Autodesk Fusion 360 part; units mm, degrees
(part 7 of 9)
  spline S37 degree 5 poles (66.3384, -8.5688) (66.3471, -8.5734) (66.3642, -8.5827) (66.3895, -8.5974) (66.4225, -8.6182) (66.4628, -8.6459) (66.5024, -8.6748) (66.5415, -8.7044) (66.5803, -8.7345) (66.6191, -8.7648) (66.6576, -8.7955) (66.6959, -8.8265) (66.7339, -8.858) (66.7716, -8.8901) (66.8088, -8.9228) (66.8458, -8.956) (66.8824, -8.9896) (66.9188, -9.0237) (66.955, -9.0581) (66.9909, -9.0927) (67.0267, -9.1277) (67.0622, -9.1631) (67.0975, -9.1987) (67.1325, -9.2348) (67.1673, -9.2712) (67.2019, -9.3079) (67.2362, -9.3449) (67.2704, -9.3822) (67.3043, -9.4198) (67.338, -9.4577) (67.3716, -9.4959) (67.4049, -9.5344) (67.438, -9.5731) (67.4709, -9.6121) (67.5036, -9.6514) (67.5361, -9.6909) (67.5684, -9.7307) (67.6005, -9.7708) (67.6324, -9.8111) (67.6641, -9.8517) (67.6956, -9.8925) (67.727, -9.9335) (67.7581, -9.9748) (67.7891, -10.0163) (67.8198, -10.0581) (67.8504, -10.1001) (67.8808, -10.1423) (67.911, -10.1847) (67.941, -10.2274) (67.9708, -10.2703) (68.0004, -10.3134) (68.0299, -10.3567) (68.0592, -10.4002) (68.0882, -10.4439) (68.1171, -10.4879) (68.1459, -10.532) (68.1744, -10.5764) (68.2028, -10.621) (68.231, -10.6657) (68.259, -10.7107) (68.2868, -10.7558) (68.3144, -10.8012) (68.3419, -10.8467) (68.3692, -10.8925) (68.3963, -10.9384) (68.4232, -10.9845) (68.4499, -11.0308) (68.4765, -11.0773) (68.5029, -11.124) (68.5291, -11.1708) (68.5551, -11.2178) (68.5758, -11.2556) (68.5913, -11.284) (68.6015, -11.303) (68.6067, -11.3125) knots 0 0 0 0 0 0 0.01428571 0.02857143 0.04285714 0.05714286 0.07142857 0.08571429 0.1 0.11428571 0.12857143 0.14285714 0.15714286 0.17142857 0.18571429 0.2 0.21428571 0.22857143 0.24285714 0.25714286 0.27142857 0.28571429 0.3 0.31428571 0.32857143 0.34285714 0.35714286 0.37142857 0.38571429 0.4 0.41428571 0.42857143 0.44285714 0.45714286 0.47142857 0.48571429 0.5 0.51428571 0.52857143 0.54285714 0.55714286 0.57142857 0.58571429 0.6 0.61428571 0.62857143 0.64285714 0.65714286 0.67142857 0.68571429 0.7 0.71428571 0.72857143 0.74285714 0.75714286 0.77142857 0.78571429 0.8 0.81428571 0.82857143 0.84285714 0.85714286 0.87142857 0.88571429 0.9 0.91428571 0.92857143 0.94285714 0.95714286 0.97142857 0.98571429 1 1 1 1 1 1
  line L37 (66.3384, -8.5688) -> (66.2067, -8.499)
  arc A75 (65.7693, -7.1913) -> (66.2067, -8.499) centre (66.6749, -7.6154) ccw
  arc A76 (65.7693, -7.1913) -> (65.9238, -6.8531) centre (48.0648, 1.0985) ccw
  arc A77 (67.1984, -6.3273) -> (65.9238, -6.8531) centre (66.8373, -7.2598) ccw
  line L38 (67.1984, -6.3273) -> (67.3375, -6.3811)
  spline S38 degree 5 poles (67.3375, -6.3811) (67.3466, -6.3847) (67.3649, -6.3915) (67.3926, -6.401) (67.4299, -6.4123) (67.4772, -6.4246) (67.5249, -6.4356) (67.573, -6.4458) (67.6211, -6.4555) (67.6694, -6.4648) (67.7178, -6.4739) (67.7664, -6.4825) (67.8151, -6.4906) (67.864, -6.4981) (67.9131, -6.5048) (67.9623, -6.511) (68.0118, -6.5167) (68.0613, -6.5219) (68.111, -6.5267) (68.1608, -6.5311) (68.2106, -6.5352) (68.2606, -6.5389) (68.3107, -6.5422) (68.3608, -6.5451) (68.4111, -6.5476) (68.4615, -6.5497) (68.512, -6.5514) (68.5626, -6.5528) (68.6132, -6.5538) (68.6639, -6.5544) (68.7147, -6.5548) (68.7656, -6.5548) (68.8166, -6.5544) (68.8676, -6.5538) (68.9187, -6.5527) (68.9699, -6.5514) (69.0211, -6.5498) (69.0724, -6.5478) (69.1238, -6.5455) (69.1752, -6.5429) (69.2267, -6.54) (69.2782, -6.5368) (69.3298, -6.5333) (69.3814, -6.5295) (69.4331, -6.5254) (69.4849, -6.521) (69.5367, -6.5163) (69.5885, -6.5114) (69.6404, -6.5061) (69.6924, -6.5006) (69.7443, -6.4947) (69.7964, -6.4886) (69.8484, -6.4822) (69.9005, -6.4756) (69.9527, -6.4687) (70.0049, -6.4614) (70.0571, -6.454) (70.1093, -6.4462) (70.1616, -6.4382) (70.2139, -6.4299) (70.2663, -6.4214) (70.3186, -6.4126) (70.371, -6.4035) (70.4235, -6.3942) (70.4759, -6.3846) (70.5284, -6.3747) (70.5809, -6.3646) (70.6334, -6.3543) (70.686, -6.3436) (70.7386, -6.3328) (70.7912, -6.3217) (70.8332, -6.3126) (70.8648, -6.3056) (70.8859, -6.301) (70.8964, -6.2986) knots 0 0 0 0 0 0 0.01428571 0.02857143 0.04285714 0.05714286 0.07142857 0.08571429 0.1 0.11428571 0.12857143 0.14285714 0.15714286 0.17142857 0.18571429 0.2 0.21428571 0.22857143 0.24285714 0.25714286 0.27142857 0.28571429 0.3 0.31428571 0.32857143 0.34285714 0.35714286 0.37142857 0.38571429 0.4 0.41428571 0.42857143 0.44285714 0.45714286 0.47142857 0.48571429 0.5 0.51428571 0.52857143 0.54285714 0.55714286 0.57142857 0.58571429 0.6 0.61428571 0.62857143 0.64285714 0.65714286 0.67142857 0.68571429 0.7 0.71428571 0.72857143 0.74285714 0.75714286 0.77142857 0.78571429 0.8 0.81428571 0.82857143 0.84285714 0.85714286 0.87142857 0.88571429 0.9 0.91428571 0.92857143 0.94285714 0.95714286 0.97142857 0.98571429 1 1 1 1 1 1
  arc A78 (70.8964, -6.2986) -> (71.2711, -5.0224) centre (48.0648, 1.0985) ccw
  spline S39 degree 5 poles (68.3218, -3.0289) (68.3314, -3.0309) (68.3505, -3.035) (68.3789, -3.042) (68.4164, -3.0526) (68.4629, -3.0678) (68.509, -3.0844) (68.5548, -3.1018) (68.6006, -3.1197) (68.6463, -3.138) (68.6919, -3.1565) (68.7374, -3.1755) (68.7828, -3.195) (68.8279, -3.2152) (68.8729, -3.236) (68.9177, -3.2575) (68.9623, -3.2794) (69.0068, -3.3019) (69.0512, -3.3247) (69.0955, -3.3478) (69.1396, -3.3713) (69.1837, -3.3952) (69.2276, -3.4195) (69.2714, -3.4442) (69.315, -3.4693) (69.3585, -3.4948) (69.4019, -3.5206) (69.4452, -3.5468) (69.4883, -3.5734) (69.5314, -3.6002) (69.5743, -3.6274) (69.6171, -3.6549) (69.6598, -3.6828) (69.7023, -3.7109) (69.7448, -3.7394) (69.7871, -3.7682) (69.8293, -3.7973) (69.8714, -3.8267) (69.9134, -3.8564) (69.9552, -3.8864) (69.997, -3.9166) (70.0386, -3.9472) (70.0801, -3.978) (70.1215, -4.0091) (70.1628, -4.0405) (70.2039, -4.0722) (70.245, -4.1042) (70.2859, -4.1364) (70.3267, -4.1688) (70.3674, -4.2016) (70.408, -4.2346) (70.4484, -4.2678) (70.4888, -4.3014) (70.529, -4.3351) (70.5691, -4.3692) (70.6091, -4.4034) (70.649, -4.438) (70.6888, -4.4727) (70.7284, -4.5077) (70.768, -4.543) (70.8074, -4.5785) (70.8467, -4.6142) (70.8859, -4.6501) (70.9249, -4.6863) (70.9639, -4.7228) (71.0027, -4.7594) (71.0414, -4.7963) (71.08, -4.8334) (71.1185, -4.8708) (71.1568, -4.9083) (71.195, -4.9461) (71.2255, -4.9765) (71.2484, -4.9994) (71.2635, -5.0148) (71.2711, -5.0224) knots 0 0 0 0 0 0 0.01428571 0.02857143 0.04285714 0.05714286 0.07142857 0.08571429 0.1 0.11428571 0.12857143 0.14285714 0.15714286 0.17142857 0.18571429 0.2 0.21428571 0.22857143 0.24285714 0.25714286 0.27142857 0.28571429 0.3 0.31428571 0.32857143 0.34285714 0.35714286 0.37142857 0.38571429 0.4 0.41428571 0.42857143 0.44285714 0.45714286 0.47142857 0.48571429 0.5 0.51428571 0.52857143 0.54285714 0.55714286 0.57142857 0.58571429 0.6 0.61428571 0.62857143 0.64285714 0.65714286 0.67142857 0.68571429 0.7 0.71428571 0.72857143 0.74285714 0.75714286 0.77142857 0.78571429 0.8 0.81428571 0.82857143 0.84285714 0.85714286 0.87142857 0.88571429 0.9 0.91428571 0.92857143 0.94285714 0.95714286 0.97142857 0.98571429 1 1 1 1 1 1
  line L39 (68.3218, -3.0289) -> (68.1757, -2.999)
  arc A79 (67.3877, -1.8676) -> (68.1757, -2.999) centre (68.3761, -2.0193) ccw
  arc A80 (67.3877, -1.8676) -> (67.4406, -1.4995) centre (48.0648, 1.0985) ccw
  arc A81 (68.5155, -0.6359) -> (67.4406, -1.4995) centre (68.4317, -1.6324) ccw
  line L40 (68.5155, -0.6359) -> (68.6641, -0.6484)
  spline S40 degree 5 poles (68.6641, -0.6484) (68.6738, -0.6492) (68.6933, -0.6506) (68.7225, -0.6519) (68.7615, -0.6523) (68.8104, -0.6508) (68.8593, -0.6479) (68.9082, -0.6441) (68.9572, -0.6398) (69.0061, -0.6352) (69.0551, -0.6303) (69.1041, -0.6249) (69.1531, -0.6189) (69.2022, -0.6123) (69.2512, -0.605) (69.3002, -0.597) (69.3492, -0.5885) (69.3982, -0.5795) (69.4472, -0.5701) (69.4962, -0.5604) (69.5452, -0.5503) (69.5942, -0.5398) (69.6432, -0.5288) (69.6922, -0.5175) (69.7411, -0.5057) (69.79, -0.4935) (69.839, -0.4809) (69.8879, -0.468) (69.9367, -0.4546) (69.9856, -0.441) (70.0344, -0.427) (70.0832, -0.4127) (70.132, -0.398) (70.1808, -0.383) (70.2296, -0.3676) (70.2783, -0.3519) (70.327, -0.3359) (70.3756, -0.3195) (70.4243, -0.3029) (70.4729, -0.2859) (70.5215, -0.2686) (70.57, -0.251) (70.6185, -0.2331) (70.667, -0.2149) (70.7155, -0.1964) (70.7639, -0.1776) (70.8123, -0.1585) (70.8606, -0.1392) (70.9089, -0.1195) (70.9572, -0.0995) (71.0054, -0.0793) (71.0536, -0.0588) (71.1018, -0.038) (71.1499, -0.0169) (71.198, 0.0044) (71.246, 0.026) (71.294, 0.0479) (71.3419, 0.0701) (71.3898, 0.0925) (71.4377, 0.1152) (71.4855, 0.1381) (71.5333, 0.1613) (71.581, 0.1848) (71.6287, 0.2085) (71.6763, 0.2325) (71.7239, 0.2567) (71.7714, 0.2812) (71.8189, 0.306) (71.8664, 0.3309) (71.9137, 0.3562) (71.9611, 0.3817) (71.9989, 0.4023) (72.0272, 0.4178) (72.0461, 0.4282) (72.0556, 0.4334) knots 0 0 0 0 0 0 0.01428571 0.02857143 0.04285714 0.05714286 0.07142857 0.08571429 0.1 0.11428571 0.12857143 0.14285714 0.15714286 0.17142857 0.18571429 0.2 0.21428571 0.22857143 0.24285714 0.25714286 0.27142857 0.28571429 0.3 0.31428571 0.32857143 0.34285714 0.35714286 0.37142857 0.38571429 0.4 0.41428571 0.42857143 0.44285714 0.45714286 0.47142857 0.48571429 0.5 0.51428571 0.52857143 0.54285714 0.55714286 0.57142857 0.58571429 0.6 0.61428571 0.62857143 0.64285714 0.65714286 0.67142857 0.68571429 0.7 0.71428571 0.72857143 0.74285714 0.75714286 0.77142857 0.78571429 0.8 0.81428571 0.82857143 0.84285714 0.85714286 0.87142857 0.88571429 0.9 0.91428571 0.92857143 0.94285714 0.95714286 0.97142857 0.98571429 1 1 1 1 1 1
  arc A82 (72.0556, 0.4334) -> (72.0556, 1.7635) centre (48.0648, 1.0985) ccw
  spline S41 degree 5 poles (68.6641, 2.8453) (68.6738, 2.8461) (68.6933, 2.8475) (68.7225, 2.8489) (68.7615, 2.8492) (68.8104, 2.8477) (68.8593, 2.8448) (68.9082, 2.841) (68.9572, 2.8367) (69.0061, 2.8321) (69.0551, 2.8272) (69.1041, 2.8218) (69.1531, 2.8159) (69.2022, 2.8092) (69.2512, 2.8019) (69.3002, 2.7939) (69.3492, 2.7854) (69.3982, 2.7764) (69.4472, 2.7671) (69.4962, 2.7573) (69.5452, 2.7472) (69.5942, 2.7367) (69.6432, 2.7257) (69.6922, 2.7144) (69.7411, 2.7026) (69.79, 2.6904) (69.839, 2.6778) (69.8879, 2.6649) (69.9367, 2.6516) (69.9856, 2.6379) (70.0344, 2.6239) (70.0832, 2.6096) (70.132, 2.5949) (70.1808, 2.5799) (70.2296, 2.5645) (70.2783, 2.5488) (70.327, 2.5328) (70.3756, 2.5165) (70.4243, 2.4998) (70.4729, 2.4828) (70.5215, 2.4655) (70.57, 2.4479) (70.6185, 2.43) (70.667, 2.4118) (70.7155, 2.3933) (70.7639, 2.3746) (70.8123, 2.3555) (70.8606, 2.3361) (70.9089, 2.3164) (70.9572, 2.2965) (71.0054, 2.2762) (71.0536, 2.2557) (71.1018, 2.2349) (71.1499, 2.2139) (71.198, 2.1925) (71.246, 2.1709) (71.294, 2.149) (71.3419, 2.1269) (71.3898, 2.1045) (71.4377, 2.0818) (71.4855, 2.0588) (71.5333, 2.0356) (71.581, 2.0122) (71.6287, 1.9884) (71.6763, 1.9644) (71.7239, 1.9402) (71.7714, 1.9157) (71.8189, 1.891) (71.8664, 1.866) (71.9137, 1.8408) (71.9611, 1.8153) (71.9989, 1.7947) (72.0272, 1.7791) (72.0461, 1.7687) (72.0556, 1.7635) knots 0 0 0 0 0 0 0.01428571 0.02857143 0.04285714 0.05714286 0.07142857 0.08571429 0.1 0.11428571 0.12857143 0.14285714 0.15714286 0.17142857 0.18571429 0.2 0.21428571 0.22857143 0.24285714 0.25714286 0.27142857 0.28571429 0.3 0.31428571 0.32857143 0.34285714 0.35714286 0.37142857 0.38571429 0.4 0.41428571 0.42857143 0.44285714 0.45714286 0.47142857 0.48571429 0.5 0.51428571 0.52857143 0.54285714 0.55714286 0.57142857 0.58571429 0.6 0.61428571 0.62857143 0.64285714 0.65714286 0.67142857 0.68571429 0.7 0.71428571 0.72857143 0.74285714 0.75714286 0.77142857 0.78571429 0.8 0.81428571 0.82857143 0.84285714 0.85714286 0.87142857 0.88571429 0.9 0.91428571 0.92857143 0.94285714 0.95714286 0.97142857 0.98571429 1 1 1 1 1 1
  line L41 (68.6641, 2.8453) -> (68.5155, 2.8328)
  arc A83 (67.4406, 3.6964) -> (68.5155, 2.8328) centre (68.4317, 3.8293) ccw
  arc A84 (67.4406, 3.6964) -> (67.3877, 4.0645) centre (48.0648, 1.0985) ccw
  arc A85 (68.1757, 5.196) -> (67.3877, 4.0645) centre (68.3761, 4.2163) ccw
  line L42 (68.1757, 5.196) -> (68.3218, 5.2259)
  spline S42 degree 5 poles (68.3218, 5.2259) (68.3314, 5.2278) (68.3505, 5.232) (68.3789, 5.2389) (68.4164, 5.2496) (68.4629, 5.2648) (68.509, 5.2814) (68.5548, 5.2988) (68.6006, 5.3167) (68.6463, 5.3349) (68.6919, 5.3534) (68.7374, 5.3724) (68.7828, 5.3919) (68.8279, 5.4121) (68.8729, 5.4329) (68.9177, 5.4544) (68.9623, 5.4764) (69.0068, 5.4988) (69.0512, 5.5216) (69.0955, 5.5447) (69.1396, 5.5683) (69.1837, 5.5922) (69.2276, 5.6164) (69.2714, 5.6411) (69.315, 5.6662) (69.3585, 5.6917) (69.4019, 5.7176) (69.4452, 5.7438) (69.4883, 5.7703) (69.5314, 5.7972) (69.5743, 5.8244) (69.6171, 5.8519) (69.6598, 5.8797) (69.7023, 5.9079) (69.7448, 5.9363) (69.7871, 5.9651) (69.8293, 5.9942) (69.8714, 6.0236) (69.9134, 6.0533) (69.9552, 6.0833) (69.997, 6.1136) (70.0386, 6.1441) (70.0801, 6.1749) (70.1215, 6.2061) (70.1628, 6.2375) (70.2039, 6.2691) (70.245, 6.3011) (70.2859, 6.3333) (70.3267, 6.3658) (70.3674, 6.3985) (70.408, 6.4315) (70.4484, 6.4648) (70.4888, 6.4983) (70.529, 6.5321) (70.5691, 6.5661) (70.6091, 6.6004) (70.649, 6.6349) (70.6888, 6.6696) (70.7284, 6.7047) (70.768, 6.7399) (70.8074, 6.7754) (70.8467, 6.8111) (70.8859, 6.8471) (70.9249, 6.8833) (70.9639, 6.9197) (71.0027, 6.9564) (71.0414, 6.9933) (71.08, 7.0304) (71.1185, 7.0677) (71.1568, 7.1053) (71.195, 7.1431) (71.2255, 7.1735) (71.2484, 7.1964) (71.2635, 7.2117) (71.2711, 7.2194) knots 0 0 0 0 0 0 0.01428571 0.02857143 0.04285714 0.05714286 0.07142857 0.08571429 0.1 0.11428571 0.12857143 0.14285714 0.15714286 0.17142857 0.18571429 0.2 0.21428571 0.22857143 0.24285714 0.25714286 0.27142857 0.28571429 0.3 0.31428571 0.32857143 0.34285714 0.35714286 0.37142857 0.38571429 0.4 0.41428571 0.42857143 0.44285714 0.45714286 0.47142857 0.48571429 0.5 0.51428571 0.52857143 0.54285714 0.55714286 0.57142857 0.58571429 0.6 0.61428571 0.62857143 0.64285714 0.65714286 0.67142857 0.68571429 0.7 0.71428571 0.72857143 0.74285714 0.75714286 0.77142857 0.78571429 0.8 0.81428571 0.82857143 0.84285714 0.85714286 0.87142857 0.88571429 0.9 0.91428571 0.92857143 0.94285714 0.95714286 0.97142857 0.98571429 1 1 1 1 1 1
  arc A86 (71.2711, 7.2194) -> (70.8964, 8.4955) centre (48.0648, 1.0985) ccw
  spline S43 degree 5 poles (67.3375, 8.5781) (67.3466, 8.5816) (67.3649, 8.5884) (67.3926, 8.5979) (67.4299, 8.6093) (67.4772, 8.6216) (67.5249, 8.6326) (67.573, 8.6427) (67.6211, 8.6524) (67.6694, 8.6618) (67.7178, 8.6708) (67.7664, 8.6795) (67.8151, 8.6876) (67.864, 8.695) (67.9131, 8.7018) (67.9623, 8.708) (68.0118, 8.7136) (68.0613, 8.7188) (68.111, 8.7236) (68.1608, 8.7281) (68.2106, 8.7322) (68.2606, 8.7359) (68.3107, 8.7392) (68.3608, 8.7421) (68.4111, 8.7446) (68.4615, 8.7466) (68.512, 8.7483) (68.5626, 8.7497) (68.6132, 8.7507) (68.6639, 8.7514) (68.7147, 8.7517) (68.7656, 8.7517) (68.8166, 8.7514) (68.8676, 8.7507) (68.9187, 8.7497) (68.9699, 8.7483) (69.0211, 8.7467) (69.0724, 8.7447) (69.1238, 8.7424) (69.1752, 8.7398) (69.2267, 8.7369) (69.2782, 8.7337) (69.3298, 8.7302) (69.3814, 8.7264) (69.4331, 8.7223) (69.4849, 8.7179) (69.5367, 8.7133) (69.5885, 8.7083) (69.6404, 8.703) (69.6924, 8.6975) (69.7443, 8.6917) (69.7964, 8.6856) (69.8484, 8.6792) (69.9005, 8.6725) (69.9527, 8.6656) (70.0049, 8.6584) (70.0571, 8.6509) (70.1093, 8.6432) (70.1616, 8.6351) (70.2139, 8.6269) (70.2663, 8.6183) (70.3186, 8.6095) (70.371, 8.6004) (70.4235, 8.5911) (70.4759, 8.5815) (70.5284, 8.5717) (70.5809, 8.5616) (70.6334, 8.5512) (70.686, 8.5406) (70.7386, 8.5297) (70.7912, 8.5186) (70.8332, 8.5095) (70.8648, 8.5026) (70.8859, 8.4979) (70.8964, 8.4955) knots 0 0 0 0 0 0 0.01428571 0.02857143 0.04285714 0.05714286 0.07142857 0.08571429 0.1 0.11428571 0.12857143 0.14285714 0.15714286 0.17142857 0.18571429 0.2 0.21428571 0.22857143 0.24285714 0.25714286 0.27142857 0.28571429 0.3 0.31428571 0.32857143 0.34285714 0.35714286 0.37142857 0.38571429 0.4 0.41428571 0.42857143 0.44285714 0.45714286 0.47142857 0.48571429 0.5 0.51428571 0.52857143 0.54285714 0.55714286 0.57142857 0.58571429 0.6 0.61428571 0.62857143 0.64285714 0.65714286 0.67142857 0.68571429 0.7 0.71428571 0.72857143 0.74285714 0.75714286 0.77142857 0.78571429 0.8 0.81428571 0.82857143 0.84285714 0.85714286 0.87142857 0.88571429 0.9 0.91428571 0.92857143 0.94285714 0.95714286 0.97142857 0.98571429 1 1 1 1 1 1
  line L43 (67.3375, 8.5781) -> (67.1984, 8.5242)
  arc A87 (65.9238, 9.05) -> (67.1984, 8.5242) centre (66.8373, 9.4567) ccw
  arc A88 (65.9238, 9.05) -> (65.7693, 9.3883) centre (48.0648, 1.0985) ccw
  circle A89 centre (48.0648, 1.0985) radius 15
  constraint concentric A0 A89
extrude "Extrude3''" add sketch "Sketch6" along normal blind 3 contours A0 A89 | A1 L0 S0 A2 S1 L1 A3 A4 A5 L2 S2 A6 S3 L3 A7 A8 A9 L4 S4 A10 S5 L5 A11 A12 A13 L6 S6 A14 S7 L7 A15 A16 A17 L8 S8 A18 S9 L9 A19 A20 A21 L10 S10 A22 S11 L11 A23 A24 A25 L12 S12 A26 S13 L13 A27 A28 A29 L14 S14 A30 S15 L15 A31 A32 A33 L16 S16 A34 S17 L17 A35 A36 A37 L18 S18 A38 S19 L19 A39 A40 A41 L20 S20 A42 S21 L21 A43 A44 A45 L22 S22 A46 S23 L23 A47 A48 A49 L24 S24 A50 S25 L25 A51 A52 A53 L26 S26 A54 S27 L27 A55 A56 A57 L28 S28 A58 S29 L29 A59 A60 A61 L30 S30 A62 S31 L31 A63 A64 A65 L32 S32 A66 S33 L33 A67 A68 A69 L34 S34 A70 S35 L35 A71 A72 A73 L36 S36 A74 S37 L37 A75 A76 A77 L38 S38 A78 S39 L39 A79 A80 A81 L40 S40 A82 S41 L41 A83 A84 A85 L42 S42 A86 S43 L43 A87 A88 sketch seen with x (1, 0, 0) y (0, 1, 0) z (0, 0, 1) at (-48.0648, 1.0985, 0.2907) bodies 2 in component "Spur Gear (22 teeth)"
sketch "Sketch7" plane through (0, 0, -0.7135) normal (0, 0, -1) x (1, 0, 0)
  circle A0 centre (-0.4607, 2.7328) radius 15
  arc A1 (15.3748, 12.1549) -> (15.0406, 10.9599) centre (15.8355, 11.3818) ccw
  line L0 (15.3748, 12.1549) -> (15.6903, 12.3429)
  spline S0 degree 5 poles (15.6903, 12.3429) (15.6984, 12.3478) (15.7144, 12.3576) (15.7381, 12.373) (15.7688, 12.3947) (15.8062, 12.4235) (15.8428, 12.4534) (15.8789, 12.484) (15.9148, 12.5151) (15.9505, 12.5464) (15.986, 12.578) (16.0213, 12.61) (16.0562, 12.6425) (16.0907, 12.6755) (16.1249, 12.709) (16.1586, 12.7431) (16.1921, 12.7776) (16.2253, 12.8125) (16.2582, 12.8477) (16.2909, 12.8832) (16.3234, 12.919) (16.3557, 12.9552) (16.3877, 12.9916) (16.4194, 13.0284) (16.4509, 13.0655) (16.4821, 13.103) (16.5131, 13.1407) (16.5439, 13.1788) (16.5744, 13.2171) (16.6048, 13.2557) (16.6349, 13.2945) (16.6647, 13.3337) (16.6944, 13.373) (16.7238, 13.4127) (16.7531, 13.4526) (16.7821, 13.4928) (16.8109, 13.5332) (16.8394, 13.5738) (16.8678, 13.6147) (16.896, 13.6559) (16.9239, 13.6972) (16.9517, 13.7388) (16.9792, 13.7807) (17.0066, 13.8227) (17.0337, 13.865) (17.0607, 13.9075) (17.0874, 13.9502) (17.1139, 13.9931) (17.1403, 14.0363) (17.1664, 14.0796) (17.1923, 14.1232) (17.2181, 14.1669) (17.2436, 14.2109) (17.269, 14.255) (17.2941, 14.2994) (17.3191, 14.344) (17.3438, 14.3887) (17.3684, 14.4336) (17.3928, 14.4788) (17.417, 14.5241) (17.441, 14.5696) (17.4648, 14.6153) (17.4884, 14.6612) (17.5118, 14.7072) (17.535, 14.7535) (17.5581, 14.7999) (17.5809, 14.8465) (17.6036, 14.8932) (17.626, 14.9401) (17.6483, 14.9873) (17.6704, 15.0345) (17.6879, 15.0725) (17.701, 15.101) (17.7096, 15.1201) (17.7139, 15.1296) knots 0 0 0 0 0 0 0.01428571 0.02857143 0.04285714 0.05714286 0.07142857 0.08571429 0.1 0.11428571 0.12857143 0.14285714 0.15714286 0.17142857 0.18571429 0.2 0.21428571 0.22857143 0.24285714 0.25714286 0.27142857 0.28571429 0.3 0.31428571 0.32857143 0.34285714 0.35714286 0.37142857 0.38571429 0.4 0.41428571 0.42857143 0.44285714 0.45714286 0.47142857 0.48571429 0.5 0.51428571 0.52857143 0.54285714 0.55714286 0.57142857 0.58571429 0.6 0.61428571 0.62857143 0.64285714 0.65714286 0.67142857 0.68571429 0.7 0.71428571 0.72857143 0.74285714 0.75714286 0.77142857 0.78571429 0.8 0.81428571 0.82857143 0.84285714 0.85714286 0.87142857 0.88571429 0.9 0.91428571 0.92857143 0.94285714 0.95714286 0.97142857 0.98571429 1 1 1 1 1 1
  arc A2 (17.7139, 15.1296) -> (16.9457, 16.1871) centre (-0.4607, 2.7328) ccw
  spline S1 degree 5 poles (13.67, 15.1236) (13.6771, 15.1298) (13.6914, 15.142) (13.7134, 15.1598) (13.7435, 15.1823) (13.7824, 15.209) (13.8222, 15.2345) (13.8625, 15.2594) (13.9031, 15.2839) (13.944, 15.3082) (13.985, 15.3322) (14.0263, 15.3558) (14.0679, 15.379) (14.11, 15.4017) (14.1525, 15.4238) (14.1953, 15.4454) (14.2385, 15.4665) (14.2819, 15.4873) (14.3256, 15.5077) (14.3695, 15.5279) (14.4136, 15.5477) (14.4579, 15.5672) (14.5025, 15.5864) (14.5473, 15.6052) (14.5923, 15.6237) (14.6376, 15.6418) (14.683, 15.6596) (14.7287, 15.6771) (14.7746, 15.6943) (14.8207, 15.7113) (14.8669, 15.7279) (14.9134, 15.7442) (14.96, 15.7602) (15.0068, 15.776) (15.0538, 15.7915) (15.101, 15.8066) (15.1483, 15.8215) (15.1958, 15.8361) (15.2435, 15.8505) (15.2913, 15.8646) (15.3393, 15.8784) (15.3874, 15.8919) (15.4357, 15.9052) (15.4841, 15.9182) (15.5327, 15.9309) (15.5815, 15.9434) (15.6303, 15.9556) (15.6794, 15.9676) (15.7285, 15.9793) (15.7778, 15.9908) (15.8273, 16.002) (15.8768, 16.013) (15.9265, 16.0237) (15.9764, 16.0341) (16.0263, 16.0444) (16.0764, 16.0543) (16.1266, 16.064) (16.177, 16.0735) (16.2274, 16.0828) (16.278, 16.0918) (16.3287, 16.1005) (16.3795, 16.109) (16.4304, 16.1173) (16.4815, 16.1253) (16.5326, 16.1331) (16.5839, 16.1407) (16.6352, 16.148) (16.6867, 16.1551) (16.7383, 16.162) (16.79, 16.1686) (16.8418, 16.175) (16.8833, 16.18) (16.9145, 16.1836) (16.9353, 16.1859) (16.9457, 16.1871) knots 0 0 0 0 0 0 0.01428571 0.02857143 0.04285714 0.05714286 0.07142857 0.08571429 0.1 0.11428571 0.12857143 0.14285714 0.15714286 0.17142857 0.18571429 0.2 0.21428571 0.22857143 0.24285714 0.25714286 0.27142857 0.28571429 0.3 0.31428571 0.32857143 0.34285714 0.35714286 0.37142857 0.38571429 0.4 0.41428571 0.42857143 0.44285714 0.45714286 0.47142857 0.48571429 0.5 0.51428571 0.52857143 0.54285714 0.55714286 0.57142857 0.58571429 0.6 0.61428571 0.62857143 0.64285714 0.65714286 0.67142857 0.68571429 0.7 0.71428571 0.72857143 0.74285714 0.75714286 0.77142857 0.78571429 0.8 0.81428571 0.82857143 0.84285714 0.85714286 0.87142857 0.88571429 0.9 0.91428571 0.92857143 0.94285714 0.95714286 0.97142857 0.98571429 1 1 1 1 1 1
  line L1 (13.67, 15.1236) -> (13.3937, 14.8816)
  arc A3 (12.1539, 14.9331) -> (13.3937, 14.8816) centre (12.8008, 15.5587) ccw
  arc A4 (12.1539, 14.9331) -> (11.7396, 15.3474) centre (-0.4607, 2.7328) ccw
  arc A5 (11.6881, 16.5872) -> (11.7396, 15.3474) centre (12.3653, 15.9943) ccw
  line L2 (11.6881, 16.5872) -> (11.9301, 16.8635)
  spline S2 degree 5 poles (11.9301, 16.8635) (11.9363, 16.8706) (11.9485, 16.8849) (11.9663, 16.9069) (11.9888, 16.937) (12.0155, 16.9759) (12.041, 17.0157) (12.0659, 17.056) (12.0904, 17.0966) (12.1147, 17.1374) (12.1387, 17.1785) (12.1623, 17.2198) (12.1855, 17.2614) (12.2082, 17.3035) (12.2303, 17.346) (12.2519, 17.3888) (12.273, 17.432) (12.2938, 17.4754) (12.3142, 17.5191) (12.3344, 17.563) (12.3542, 17.6071) (12.3737, 17.6514) (12.3929, 17.6959) (12.4117, 17.7407) (12.4302, 17.7858) (12.4483, 17.8311) (12.4661, 17.8765) (12.4836, 17.9222) (12.5008, 17.9681) (12.5178, 18.0142) (12.5344, 18.0604) (12.5507, 18.1069) (12.5668, 18.1535) (12.5825, 18.2003) (12.598, 18.2473) (12.6131, 18.2944) (12.628, 18.3418) (12.6426, 18.3893) (12.657, 18.4369) (12.6711, 18.4848) (12.6849, 18.5328) (12.6984, 18.5809) (12.7117, 18.6292) (12.7247, 18.6776) (12.7374, 18.7262) (12.7499, 18.775) (12.7622, 18.8238) (12.7741, 18.8729) (12.7858, 18.922) (12.7973, 18.9713) (12.8085, 19.0208) (12.8195, 19.0703) (12.8302, 19.12) (12.8406, 19.1699) (12.8509, 19.2198) (12.8608, 19.2699) (12.8706, 19.3201) (12.88, 19.3705) (12.8893, 19.4209) (12.8983, 19.4715) (12.907, 19.5222) (12.9155, 19.573) (12.9238, 19.6239) (12.9319, 19.675) (12.9397, 19.7261) (12.9472, 19.7774) (12.9545, 19.8287) (12.9616, 19.8802) (12.9685, 19.9318) (12.9751, 19.9835) (12.9815, 20.0353) (12.9865, 20.0768) (12.9901, 20.1079) (12.9924, 20.1288) (12.9936, 20.1392) knots 0 0 0 0 0 0 0.01428571 0.02857143 0.04285714 0.05714286 0.07142857 0.08571429 0.1 0.11428571 0.12857143 0.14285714 0.15714286 0.17142857 0.18571429 0.2 0.21428571 0.22857143 0.24285714 0.25714286 0.27142857 0.28571429 0.3 0.31428571 0.32857143 0.34285714 0.35714286 0.37142857 0.38571429 0.4 0.41428571 0.42857143 0.44285714 0.45714286 0.47142857 0.48571429 0.5 0.51428571 0.52857143 0.54285714 0.55714286 0.57142857 0.58571429 0.6 0.61428571 0.62857143 0.64285714 0.65714286 0.67142857 0.68571429 0.7 0.71428571 0.72857143 0.74285714 0.75714286 0.77142857 0.78571429 0.8 0.81428571 0.82857143 0.84285714 0.85714286 0.87142857 0.88571429 0.9 0.91428571 0.92857143 0.94285714 0.95714286 0.97142857 0.98571429 1 1 1 1 1 1
  arc A6 (12.9936, 20.1392) -> (11.9361, 20.9074) centre (-0.4607, 2.7328) ccw
  spline S3 degree 5 poles (9.1494, 18.8838) (9.1543, 18.8919) (9.1641, 18.9079) (9.1795, 18.9316) (9.2012, 18.9623) (9.23, 18.9997) (9.2599, 19.0363) (9.2905, 19.0724) (9.3216, 19.1083) (9.3529, 19.144) (9.3845, 19.1795) (9.4165, 19.2148) (9.449, 19.2497) (9.482, 19.2842) (9.5155, 19.3184) (9.5496, 19.3521) (9.5841, 19.3856) (9.619, 19.4188) (9.6542, 19.4517) (9.6897, 19.4844) (9.7255, 19.5169) (9.7617, 19.5492) (9.7981, 19.5812) (9.8349, 19.6129) (9.872, 19.6444) (9.9095, 19.6756) (9.9472, 19.7066) (9.9853, 19.7374) (10.0236, 19.7679) (10.0622, 19.7983) (10.101, 19.8284) (10.1402, 19.8582) (10.1795, 19.8879) (10.2192, 19.9173) (10.2591, 19.9466) (10.2993, 19.9756) (10.3397, 20.0044) (10.3803, 20.0329) (10.4212, 20.0613) (10.4624, 20.0895) (10.5037, 20.1174) (10.5453, 20.1452) (10.5872, 20.1727) (10.6292, 20.2001) (10.6715, 20.2272) (10.714, 20.2541) (10.7567, 20.2809) (10.7996, 20.3074) (10.8428, 20.3338) (10.8861, 20.3599) (10.9297, 20.3858) (10.9734, 20.4116) (11.0174, 20.4371) (11.0615, 20.4625) (11.1059, 20.4876) (11.1505, 20.5126) (11.1952, 20.5373) (11.2402, 20.5619) (11.2853, 20.5863) (11.3306, 20.6105) (11.3761, 20.6345) (11.4218, 20.6583) (11.4677, 20.6819) (11.5137, 20.7053) (11.56, 20.7285) (11.6064, 20.7515) (11.653, 20.7744) (11.6997, 20.797) (11.7467, 20.8195) (11.7938, 20.8418) (11.841, 20.8639) (11.879, 20.8814) (11.9075, 20.8944) (11.9266, 20.9031) (11.9361, 20.9074) knots 0 0 0 0 0 0 0.01428571 0.02857143 0.04285714 0.05714286 0.07142857 0.08571429 0.1 0.11428571 0.12857143 0.14285714 0.15714286 0.17142857 0.18571429 0.2 0.21428571 0.22857143 0.24285714 0.25714286 0.27142857 0.28571429 0.3 0.31428571 0.32857143 0.34285714 0.35714286 0.37142857 0.38571429 0.4 0.41428571 0.42857143 0.44285714 0.45714286 0.47142857 0.48571429 0.5 0.51428571 0.52857143 0.54285714 0.55714286 0.57142857 0.58571429 0.6 0.61428571 0.62857143 0.64285714 0.65714286 0.67142857 0.68571429 0.7 0.71428571 0.72857143 0.74285714 0.75714286 0.77142857 0.78571429 0.8 0.81428571 0.82857143 0.84285714 0.85714286 0.87142857 0.88571429 0.9 0.91428571 0.92857143 0.94285714 0.95714286 0.97142857 0.98571429 1 1 1 1 1 1
  line L3 (9.1494, 18.8838) -> (8.9614, 18.5683)
  arc A7 (7.7664, 18.2341) -> (8.9614, 18.5683) centre (8.1883, 19.029) ccw
  arc A8 (7.7664, 18.2341) -> (7.2443, 18.5001) centre (-0.4607, 2.7328) ccw
  arc A9 (6.8123, 19.6633) -> (7.2443, 18.5001) centre (7.6395, 19.3087) ccw
  line L4 (6.8123, 19.6633) -> (6.957, 20.0009)
  spline S4 degree 5 poles (6.957, 20.0009) (6.9607, 20.0095) (6.9679, 20.0269) (6.978, 20.0533) (6.9901, 20.0889) (7.0035, 20.1342) (7.0155, 20.1799) (7.0267, 20.2259) (7.0375, 20.2721) (7.0479, 20.3184) (7.0581, 20.3649) (7.0678, 20.4115) (7.077, 20.4583) (7.0855, 20.5053) (7.0934, 20.5525) (7.1007, 20.5999) (7.1075, 20.6475) (7.1138, 20.6952) (7.1198, 20.7431) (7.1254, 20.791) (7.1306, 20.8391) (7.1355, 20.8873) (7.1399, 20.9356) (7.144, 20.984) (7.1476, 21.0326) (7.1509, 21.0812) (7.1538, 21.13) (7.1563, 21.1788) (7.1585, 21.2278) (7.1603, 21.2768) (7.1619, 21.3259) (7.163, 21.3752) (7.1639, 21.4245) (7.1644, 21.4738) (7.1646, 21.5233) (7.1644, 21.5728) (7.164, 21.6225) (7.1632, 21.6722) (7.1621, 21.7219) (7.1607, 21.7718) (7.159, 21.8217) (7.157, 21.8716) (7.1547, 21.9217) (7.1521, 21.9717) (7.1492, 22.0219) (7.146, 22.0721) (7.1426, 22.1224) (7.1388, 22.1727) (7.1348, 22.2231) (7.1304, 22.2735) (7.1258, 22.324) (7.1209, 22.3745) (7.1157, 22.4251) (7.1103, 22.4757) (7.1046, 22.5264) (7.0986, 22.5771) (7.0923, 22.6279) (7.0858, 22.6787) (7.079, 22.7295) (7.0719, 22.7804) (7.0645, 22.8313) (7.0569, 22.8823) (7.0491, 22.9333) (7.041, 22.9843) (7.0326, 23.0353) (7.0239, 23.0864) (7.015, 23.1375) (7.0059, 23.1887) (6.9964, 23.2399) (6.9868, 23.2911) (6.9769, 23.3423) (6.9687, 23.3833) (6.9625, 23.4141) (6.9583, 23.4346) (6.9562, 23.4448) knots 0 0 0 0 0 0 0.01428571 0.02857143 0.04285714 0.05714286 0.07142857 0.08571429 0.1 0.11428571 0.12857143 0.14285714 0.15714286 0.17142857 0.18571429 0.2 0.21428571 0.22857143 0.24285714 0.25714286 0.27142857 0.28571429 0.3 0.31428571 0.32857143 0.34285714 0.35714286 0.37142857 0.38571429 0.4 0.41428571 0.42857143 0.44285714 0.45714286 0.47142857 0.48571429 0.5 0.51428571 0.52857143 0.54285714 0.55714286 0.57142857 0.58571429 0.6 0.61428571 0.62857143 0.64285714 0.65714286 0.67142857 0.68571429 0.7 0.71428571 0.72857143 0.74285714 0.75714286 0.77142857 0.78571429 0.8 0.81428571 0.82857143 0.84285714 0.85714286 0.87142857 0.88571429 0.9 0.91428571 0.92857143 0.94285714 0.95714286 0.97142857 0.98571429 1 1 1 1 1 1
  arc A10 (6.9562, 23.4448) -> (5.7131, 23.8487) centre (-0.4607, 2.7328) ccw
  spline S5 degree 5 poles (3.6882, 21.063) (3.6902, 21.0722) (3.6947, 21.0905) (3.702, 21.1177) (3.7131, 21.1537) (3.7289, 21.1981) (3.7461, 21.2422) (3.764, 21.286) (3.7825, 21.3297) (3.8013, 21.3733) (3.8204, 21.4169) (3.8399, 21.4603) (3.8599, 21.5035) (3.8807, 21.5466) (3.902, 21.5894) (3.924, 21.6321) (3.9465, 21.6746) (3.9694, 21.7169) (3.9927, 21.7591) (4.0164, 21.8012) (4.0404, 21.8432) (4.0648, 21.885) (4.0896, 21.9267) (4.1148, 21.9683) (4.1403, 22.0097) (4.1663, 22.051) (4.1926, 22.0921) (4.2193, 22.1331) (4.2463, 22.174) (4.2736, 22.2148) (4.3013, 22.2554) (4.3293, 22.2959) (4.3576, 22.3363) (4.3862, 22.3765) (4.4151, 22.4167) (4.4443, 22.4567) (4.4739, 22.4965) (4.5037, 22.5363) (4.5338, 22.5759) (4.5642, 22.6154) (4.595, 22.6548) (4.6259, 22.694) (4.6572, 22.7331) (4.6887, 22.7721) (4.7206, 22.811) (4.7527, 22.8498) (4.785, 22.8884) (4.8176, 22.9269) (4.8505, 22.9653) (4.8837, 23.0035) (4.9171, 23.0416) (4.9508, 23.0797) (4.9847, 23.1175) (5.0188, 23.1553) (5.0532, 23.1929) (5.0879, 23.2304) (5.1228, 23.2678) (5.158, 23.3051) (5.1934, 23.3422) (5.229, 23.3792) (5.2648, 23.4161) (5.3009, 23.4528) (5.3373, 23.4895) (5.3738, 23.526) (5.4106, 23.5623) (5.4477, 23.5986) (5.4849, 23.6347) (5.5224, 23.6707) (5.5601, 23.7066) (5.598, 23.7423) (5.6361, 23.7779) (5.6668, 23.8063) (5.6899, 23.8276) (5.7054, 23.8417) (5.7131, 23.8487) knots 0 0 0 0 0 0 0.01428571 0.02857143 0.04285714 0.05714286 0.07142857 0.08571429 0.1 0.11428571 0.12857143 0.14285714 0.15714286 0.17142857 0.18571429 0.2 0.21428571 0.22857143 0.24285714 0.25714286 0.27142857 0.28571429 0.3 0.31428571 0.32857143 0.34285714 0.35714286 0.37142857 0.38571429 0.4 0.41428571 0.42857143 0.44285714 0.45714286 0.47142857 0.48571429 0.5 0.51428571 0.52857143 0.54285714 0.55714286 0.57142857 0.58571429 0.6 0.61428571 0.62857143 0.64285714 0.65714286 0.67142857 0.68571429 0.7 0.71428571 0.72857143 0.74285714 0.75714286 0.77142857 0.78571429 0.8 0.81428571 0.82857143 0.84285714 0.85714286 0.87142857 0.88571429 0.9 0.91428571 0.92857143 0.94285714 0.95714286 0.97142857 0.98571429 1 1 1 1 1 1
  line L5 (3.6882, 21.063) -> (3.6068, 20.7048)
  arc A11 (2.5736, 20.0177) -> (3.6068, 20.7048) centre (2.7292, 20.9041) ccw
  arc A12 (2.5736, 20.0177) -> (1.9949, 20.1093) centre (-0.4607, 2.7328) ccw
  arc A13 (1.2245, 21.0821) -> (1.9949, 20.1093) centre (2.1208, 21.0005) ccw
  line L6 (1.2245, 21.0821) -> (1.2578, 21.4479)
  spline S6 degree 5 poles (1.2578, 21.4479) (1.2587, 21.4573) (1.2601, 21.4761) (1.2616, 21.5043) (1.2621, 21.5419) (1.2608, 21.589) (1.2581, 21.6362) (1.2546, 21.6835) (1.2505, 21.7307) (1.2462, 21.778) (1.2415, 21.8253) (1.2363, 21.8727) (1.2306, 21.92) (1.2242, 21.9673) (1.2171, 22.0147) (1.2094, 22.062) (1.2011, 22.1094) (1.1924, 22.1567) (1.1833, 22.2041) (1.1738, 22.2514) (1.1639, 22.2988) (1.1536, 22.3461) (1.143, 22.3934) (1.1319, 22.4407) (1.1203, 22.488) (1.1084, 22.5353) (1.0961, 22.5826) (1.0834, 22.6298) (1.0703, 22.677) (1.0569, 22.7242) (1.0432, 22.7714) (1.0291, 22.8186) (1.0147, 22.8657) (0.9999, 22.9129) (0.9848, 22.96) (0.9693, 23.007) (0.9536, 23.0541) (0.9375, 23.1011) (0.9211, 23.1481) (0.9043, 23.1951) (0.8873, 23.242) (0.87, 23.2889) (0.8523, 23.3358) (0.8344, 23.3826) (0.8161, 23.4294) (0.7976, 23.4762) (0.7787, 23.5229) (0.7596, 23.5696) (0.7402, 23.6163) (0.7205, 23.6629) (0.7005, 23.7095) (0.6802, 23.756) (0.6597, 23.8025) (0.6388, 23.849) (0.6177, 23.8954) (0.5964, 23.9418) (0.5747, 23.9882) (0.5528, 24.0344) (0.5306, 24.0807) (0.5082, 24.1269) (0.4854, 24.1731) (0.4625, 24.2192) (0.4392, 24.2652) (0.4157, 24.3112) (0.392, 24.3572) (0.368, 24.4031) (0.3437, 24.449) (0.3192, 24.4948) (0.2944, 24.5406) (0.2694, 24.5863) (0.2442, 24.6319) (0.2237, 24.6684) (0.2083, 24.6958) (0.198, 24.714) (0.1928, 24.7231) knots 0 0 0 0 0 0 0.01428571 0.02857143 0.04285714 0.05714286 0.07142857 0.08571429 0.1 0.11428571 0.12857143 0.14285714 0.15714286 0.17142857 0.18571429 0.2 0.21428571 0.22857143 0.24285714 0.25714286 0.27142857 0.28571429 0.3 0.31428571 0.32857143 0.34285714 0.35714286 0.37142857 0.38571429 0.4 0.41428571 0.42857143 0.44285714 0.45714286 0.47142857 0.48571429 0.5 0.51428571 0.52857143 0.54285714 0.55714286 0.57142857 0.58571429 0.6 0.61428571 0.62857143 0.64285714 0.65714286 0.67142857 0.68571429 0.7 0.71428571 0.72857143 0.74285714 0.75714286 0.77142857 0.78571429 0.8 0.81428571 0.82857143 0.84285714 0.85714286 0.87142857 0.88571429 0.9 0.91428571 0.92857143 0.94285714 0.95714286 0.97142857 0.98571429 1 1 1 1 1 1
  arc A14 (0.1928, 24.7231) -> (-1.1142, 24.7231) centre (-0.4607, 2.7328) ccw
  spline S7 degree 5 poles (-2.1792, 21.4479) (-2.1801, 21.4573) (-2.1816, 21.4761) (-2.183, 21.5043) (-2.1835, 21.5419) (-2.1822, 21.589) (-2.1796, 21.6362) (-2.176, 21.6835) (-2.1719, 21.7307) (-2.1676, 21.778) (-2.1629, 21.8253) (-2.1577, 21.8727) (-2.152, 21.92) (-2.1456, 21.9673) (-2.1385, 22.0147) (-2.1308, 22.062) (-2.1225, 22.1094) (-2.1138, 22.1567) (-2.1047, 22.2041) (-2.0952, 22.2514) (-2.0853, 22.2988) (-2.0751, 22.3461) (-2.0644, 22.3934) (-2.0533, 22.4407) (-2.0417, 22.488) (-2.0298, 22.5353) (-2.0175, 22.5826) (-2.0048, 22.6298) (-1.9917, 22.677) (-1.9783, 22.7242) (-1.9646, 22.7714) (-1.9505, 22.8186) (-1.9361, 22.8657) (-1.9213, 22.9129) (-1.9062, 22.96) (-1.8908, 23.007) (-1.875, 23.0541) (-1.8589, 23.1011) (-1.8425, 23.1481) (-1.8258, 23.1951) (-1.8087, 23.242) (-1.7914, 23.2889) (-1.7737, 23.3358) (-1.7558, 23.3826) (-1.7375, 23.4294) (-1.719, 23.4762) (-1.7002, 23.5229) (-1.681, 23.5696) (-1.6616, 23.6163) (-1.6419, 23.6629) (-1.6219, 23.7095) (-1.6016, 23.756) (-1.5811, 23.8025) (-1.5603, 23.849) (-1.5392, 23.8954) (-1.5178, 23.9418) (-1.4961, 23.9882) (-1.4742, 24.0344) (-1.452, 24.0807) (-1.4296, 24.1269) (-1.4069, 24.1731) (-1.3839, 24.2192) (-1.3607, 24.2652) (-1.3372, 24.3112) (-1.3134, 24.3572) (-1.2894, 24.4031) (-1.2651, 24.449) (-1.2406, 24.4948) (-1.2159, 24.5406) (-1.1908, 24.5863) (-1.1656, 24.6319) (-1.1452, 24.6684) (-1.1298, 24.6958) (-1.1194, 24.714) (-1.1142, 24.7231) knots 0 0 0 0 0 0 0.01428571 0.02857143 0.04285714 0.05714286 0.07142857 0.08571429 0.1 0.11428571 0.12857143 0.14285714 0.15714286 0.17142857 0.18571429 0.2 0.21428571 0.22857143 0.24285714 0.25714286 0.27142857 0.28571429 0.3 0.31428571 0.32857143 0.34285714 0.35714286 0.37142857 0.38571429 0.4 0.41428571 0.42857143 0.44285714 0.45714286 0.47142857 0.48571429 0.5 0.51428571 0.52857143 0.54285714 0.55714286 0.57142857 0.58571429 0.6 0.61428571 0.62857143 0.64285714 0.65714286 0.67142857 0.68571429 0.7 0.71428571 0.72857143 0.74285714 0.75714286 0.77142857 0.78571429 0.8 0.81428571 0.82857143 0.84285714 0.85714286 0.87142857 0.88571429 0.9 0.91428571 0.92857143 0.94285714 0.95714286 0.97142857 0.98571429 1 1 1 1 1 1
  line L7 (-2.1792, 21.4479) -> (-2.1459, 21.0821)
  arc A15 (-2.9163, 20.1093) -> (-2.1459, 21.0821) centre (-3.0422, 21.0005) ccw
  arc A16 (-2.9163, 20.1093) -> (-3.495, 20.0177) centre (-0.4607, 2.7328) ccw
  arc A17 (-4.5282, 20.7048) -> (-3.495, 20.0177) centre (-3.6506, 20.9041) ccw
  line L8 (-4.5282, 20.7048) -> (-4.6096, 21.063)
  spline S8 degree 5 poles (-4.6096, 21.063) (-4.6117, 21.0722) (-4.6161, 21.0905) (-4.6234, 21.1177) (-4.6346, 21.1537) (-4.6503, 21.1981) (-4.6675, 21.2422) (-4.6855, 21.286) (-4.7039, 21.3297) (-4.7227, 21.3733) (-4.7418, 21.4169) (-4.7613, 21.4603) (-4.7814, 21.5035) (-4.8021, 21.5466) (-4.8235, 21.5894) (-4.8454, 21.6321) (-4.8679, 21.6746) (-4.8909, 21.7169) (-4.9142, 21.7591) (-4.9378, 21.8012) (-4.9618, 21.8432) (-4.9862, 21.885) (-5.011, 21.9267) (-5.0362, 21.9683) (-5.0618, 22.0097) (-5.0877, 22.051) (-5.1141, 22.0921) (-5.1407, 22.1331) (-5.1677, 22.174) (-5.1951, 22.2148) (-5.2227, 22.2554) (-5.2507, 22.2959) (-5.279, 22.3363) (-5.3076, 22.3765) (-5.3365, 22.4167) (-5.3658, 22.4567) (-5.3953, 22.4965) (-5.4251, 22.5363) (-5.4553, 22.5759) (-5.4857, 22.6154) (-5.5164, 22.6548) (-5.5474, 22.694) (-5.5786, 22.7331) (-5.6102, 22.7721) (-5.642, 22.811) (-5.6741, 22.8498) (-5.7064, 22.8884) (-5.7391, 22.9269) (-5.772, 22.9653) (-5.8051, 23.0035) (-5.8385, 23.0416) (-5.8722, 23.0797) (-5.9061, 23.1175) (-5.9403, 23.1553) (-5.9747, 23.1929) (-6.0093, 23.2304) (-6.0442, 23.2678) (-6.0794, 23.3051) (-6.1148, 23.3422) (-6.1504, 23.3792) (-6.1863, 23.4161) (-6.2224, 23.4528) (-6.2587, 23.4895) (-6.2953, 23.526) (-6.3321, 23.5623) (-6.3691, 23.5986) (-6.4063, 23.6347) (-6.4438, 23.6707) (-6.4815, 23.7066) (-6.5194, 23.7423) (-6.5576, 23.7779) (-6.5882, 23.8063) (-6.6113, 23.8276) (-6.6268, 23.8417) (-6.6345, 23.8487) knots 0 0 0 0 0 0 0.01428571 0.02857143 0.04285714 0.05714286 0.07142857 0.08571429 0.1 0.11428571 0.12857143 0.14285714 0.15714286 0.17142857 0.18571429 0.2 0.21428571 0.22857143 0.24285714 0.25714286 0.27142857 0.28571429 0.3 0.31428571 0.32857143 0.34285714 0.35714286 0.37142857 0.38571429 0.4 0.41428571 0.42857143 0.44285714 0.45714286 0.47142857 0.48571429 0.5 0.51428571 0.52857143 0.54285714 0.55714286 0.57142857 0.58571429 0.6 0.61428571 0.62857143 0.64285714 0.65714286 0.67142857 0.68571429 0.7 0.71428571 0.72857143 0.74285714 0.75714286 0.77142857 0.78571429 0.8 0.81428571 0.82857143 0.84285714 0.85714286 0.87142857 0.88571429 0.9 0.91428571 0.92857143 0.94285714 0.95714286 0.97142857 0.98571429 1 1 1 1 1 1
  arc A18 (-6.6345, 23.8487) -> (-7.8776, 23.4448) centre (-0.4607, 2.7328) ccw
  spline S9 degree 5 poles (-7.8784, 20.0009) (-7.8821, 20.0095) (-7.8893, 20.0269) (-7.8994, 20.0533) (-7.9116, 20.0889) (-7.9249, 20.1342) (-7.9369, 20.1799) (-7.9481, 20.2259) (-7.9589, 20.2721) (-7.9693, 20.3184) (-7.9795, 20.3649) (-7.9892, 20.4115) (-7.9984, 20.4583) (-8.0069, 20.5053) (-8.0148, 20.5525) (-8.0221, 20.5999) (-8.0289, 20.6475) (-8.0352, 20.6952) (-8.0412, 20.7431) (-8.0468, 20.791) (-8.052, 20.8391) (-8.0569, 20.8873) (-8.0614, 20.9356) (-8.0654, 20.984) (-8.0691, 21.0326) (-8.0723, 21.0812) (-8.0752, 21.13) (-8.0777, 21.1788) (-8.0799, 21.2278) (-8.0818, 21.2768) (-8.0833, 21.3259) (-8.0845, 21.3752) (-8.0853, 21.4245) (-8.0858, 21.4738) (-8.086, 21.5233) (-8.0859, 21.5728) (-8.0854, 21.6225) (-8.0846, 21.6722) (-8.0835, 21.7219) (-8.0821, 21.7718) (-8.0804, 21.8217) (-8.0784, 21.8716) (-8.0761, 21.9217) (-8.0736, 21.9717) (-8.0707, 22.0219) (-8.0675, 22.0721) (-8.064, 22.1224) (-8.0602, 22.1727) (-8.0562, 22.2231) (-8.0518, 22.2735) (-8.0472, 22.324) (-8.0423, 22.3745) (-8.0372, 22.4251) (-8.0317, 22.4757) (-8.026, 22.5264) (-8.02, 22.5771) (-8.0137, 22.6279) (-8.0072, 22.6787) (-8.0004, 22.7295) (-7.9933, 22.7804) (-7.986, 22.8313) (-7.9784, 22.8823) (-7.9705, 22.9333) (-7.9624, 22.9843) (-7.954, 23.0353) (-7.9453, 23.0864) (-7.9364, 23.1375) (-7.9273, 23.1887) (-7.9179, 23.2399) (-7.9082, 23.2911) (-7.8983, 23.3423) (-7.8902, 23.3833) (-7.8839, 23.4141) (-7.8797, 23.4346) (-7.8776, 23.4448) knots 0 0 0 0 0 0 0.01428571 0.02857143 0.04285714 0.05714286 0.07142857 0.08571429 0.1 0.11428571 0.12857143 0.14285714 0.15714286 0.17142857 0.18571429 0.2 0.21428571 0.22857143 0.24285714 0.25714286 0.27142857 0.28571429 0.3 0.31428571 0.32857143 0.34285714 0.35714286 0.37142857 0.38571429 0.4 0.41428571 0.42857143 0.44285714 0.45714286 0.47142857 0.48571429 0.5 0.51428571 0.52857143 0.54285714 0.55714286 0.57142857 0.58571429 0.6 0.61428571 0.62857143 0.64285714 0.65714286 0.67142857 0.68571429 0.7 0.71428571 0.72857143 0.74285714 0.75714286 0.77142857 0.78571429 0.8 0.81428571 0.82857143 0.84285714 0.85714286 0.87142857 0.88571429 0.9 0.91428571 0.92857143 0.94285714 0.95714286 0.97142857 0.98571429 1 1 1 1 1 1
  line L9 (-7.8784, 20.0009) -> (-7.7337, 19.6633)
  arc A19 (-8.1657, 18.5001) -> (-7.7337, 19.6633) centre (-8.5609, 19.3087) ccw
  arc A20 (-8.1657, 18.5001) -> (-8.6878, 18.2341) centre (-0.4607, 2.7328) ccw
  arc A21 (-9.8828, 18.5683) -> (-8.6878, 18.2341) centre (-9.1097, 19.029) ccw
  line L10 (-9.8828, 18.5683) -> (-10.0709, 18.8838)
  spline S10 degree 5 poles (-10.0709, 18.8838) (-10.0757, 18.8919) (-10.0855, 18.9079) (-10.1009, 18.9316) (-10.1227, 18.9623) (-10.1514, 18.9997) (-10.1813, 19.0363) (-10.212, 19.0724) (-10.243, 19.1083) (-10.2743, 19.144) (-10.306, 19.1795) (-10.3379, 19.2148) (-10.3704, 19.2497) (-10.4034, 19.2842) (-10.437, 19.3184) (-10.471, 19.3521) (-10.5056, 19.3856) (-10.5404, 19.4188) (-10.5757, 19.4517) (-10.6112, 19.4844) (-10.647, 19.5169) (-10.6831, 19.5492) (-10.7195, 19.5812) (-10.7563, 19.6129) (-10.7935, 19.6444) (-10.8309, 19.6756) (-10.8687, 19.7066) (-10.9067, 19.7374) (-10.945, 19.7679) (-10.9836, 19.7983) (-11.0225, 19.8284) (-11.0616, 19.8582) (-11.101, 19.8879) (-11.1406, 19.9173) (-11.1805, 19.9466) (-11.2207, 19.9756) (-11.2611, 20.0044) (-11.3018, 20.0329) (-11.3427, 20.0613) (-11.3838, 20.0895) (-11.4252, 20.1174) (-11.4668, 20.1452) (-11.5086, 20.1727) (-11.5506, 20.2001) (-11.5929, 20.2272) (-11.6354, 20.2541) (-11.6781, 20.2809) (-11.7211, 20.3074) (-11.7642, 20.3338) (-11.8075, 20.3599) (-11.8511, 20.3858) (-11.8948, 20.4116) (-11.9388, 20.4371) (-11.983, 20.4625) (-12.0273, 20.4876) (-12.0719, 20.5126) (-12.1166, 20.5373) (-12.1616, 20.5619) (-12.2067, 20.5863) (-12.252, 20.6105) (-12.2975, 20.6345) (-12.3432, 20.6583) (-12.3891, 20.6819) (-12.4352, 20.7053) (-12.4814, 20.7285) (-12.5278, 20.7515) (-12.5744, 20.7744) (-12.6211, 20.797) (-12.6681, 20.8195) (-12.7152, 20.8418) (-12.7625, 20.8639) (-12.8004, 20.8814) (-12.829, 20.8944) (-12.848, 20.9031) (-12.8576, 20.9074) knots 0 0 0 0 0 0 0.01428571 0.02857143 0.04285714 0.05714286 0.07142857 0.08571429 0.1 0.11428571 0.12857143 0.14285714 0.15714286 0.17142857 0.18571429 0.2 0.21428571 0.22857143 0.24285714 0.25714286 0.27142857 0.28571429 0.3 0.31428571 0.32857143 0.34285714 0.35714286 0.37142857 0.38571429 0.4 0.41428571 0.42857143 0.44285714 0.45714286 0.47142857 0.48571429 0.5 0.51428571 0.52857143 0.54285714 0.55714286 0.57142857 0.58571429 0.6 0.61428571 0.62857143 0.64285714 0.65714286 0.67142857 0.68571429 0.7 0.71428571 0.72857143 0.74285714 0.75714286 0.77142857 0.78571429 0.8 0.81428571 0.82857143 0.84285714 0.85714286 0.87142857 0.88571429 0.9 0.91428571 0.92857143 0.94285714 0.95714286 0.97142857 0.98571429 1 1 1 1 1 1
  arc A22 (-12.8576, 20.9074) -> (-13.915, 20.1392) centre (-0.4607, 2.7328) ccw
  spline S11 degree 5 poles (-12.8515, 16.8635) (-12.8577, 16.8706) (-12.8699, 16.8849) (-12.8877, 16.9069) (-12.9102, 16.937) (-12.9369, 16.9759) (-12.9625, 17.0157) (-12.9873, 17.056) (-13.0119, 17.0966) (-13.0361, 17.1374) (-13.0601, 17.1785) (-13.0838, 17.2198) (-13.107, 17.2614) (-13.1296, 17.3035) (-13.1517, 17.346) (-13.1733, 17.3888) (-13.1944, 17.432) (-13.2152, 17.4754) (-13.2357, 17.5191) (-13.2558, 17.563) (-13.2757, 17.6071) (-13.2952, 17.6514) (-13.3143, 17.6959) (-13.3332, 17.7407) (-13.3516, 17.7858) (-13.3698, 17.8311) (-13.3876, 17.8765) (-13.4051, 17.9222) (-13.4223, 17.9681) (-13.4392, 18.0142) (-13.4558, 18.0604) (-13.4721, 18.1069) (-13.4882, 18.1535) (-13.5039, 18.2003) (-13.5194, 18.2473) (-13.5346, 18.2944) (-13.5495, 18.3418) (-13.5641, 18.3893) (-13.5784, 18.4369) (-13.5925, 18.4848) (-13.6063, 18.5328) (-13.6198, 18.5809) (-13.6331, 18.6292) (-13.6461, 18.6776) (-13.6589, 18.7262) (-13.6714, 18.775) (-13.6836, 18.8238) (-13.6956, 18.8729) (-13.7073, 18.922) (-13.7187, 18.9713) (-13.7299, 19.0208) (-13.7409, 19.0703) (-13.7516, 19.12) (-13.7621, 19.1699) (-13.7723, 19.2198) (-13.7823, 19.2699) (-13.792, 19.3201) (-13.8015, 19.3705) (-13.8107, 19.4209) (-13.8197, 19.4715) (-13.8284, 19.5222) (-13.837, 19.573) (-13.8452, 19.6239) (-13.8533, 19.675) (-13.8611, 19.7261) (-13.8686, 19.7774) (-13.876, 19.8287) (-13.8831, 19.8802) (-13.8899, 19.9318) (-13.8966, 19.9835) (-13.903, 20.0353) (-13.9079, 20.0768) (-13.9115, 20.1079) (-13.9138, 20.1288) (-13.915, 20.1392) knots 0 0 0 0 0 0 0.01428571 0.02857143 0.04285714 0.05714286 0.07142857 0.08571429 0.1 0.11428571 0.12857143 0.14285714 0.15714286 0.17142857 0.18571429 0.2 0.21428571 0.22857143 0.24285714 0.25714286 0.27142857 0.28571429 0.3 0.31428571 0.32857143 0.34285714 0.35714286 0.37142857 0.38571429 0.4 0.41428571 0.42857143 0.44285714 0.45714286 0.47142857 0.48571429 0.5 0.51428571 0.52857143 0.54285714 0.55714286 0.57142857 0.58571429 0.6 0.61428571 0.62857143 0.64285714 0.65714286 0.67142857 0.68571429 0.7 0.71428571 0.72857143 0.74285714 0.75714286 0.77142857 0.78571429 0.8 0.81428571 0.82857143 0.84285714 0.85714286 0.87142857 0.88571429 0.9 0.91428571 0.92857143 0.94285714 0.95714286 0.97142857 0.98571429 1 1 1 1 1 1
  line L11 (-12.8515, 16.8635) -> (-12.6096, 16.5872)
  arc A23 (-12.661, 15.3474) -> (-12.6096, 16.5872) centre (-13.2867, 15.9943) ccw
  arc A24 (-12.661, 15.3474) -> (-13.0753, 14.9331) centre (-0.4607, 2.7328) ccw
  arc A25 (-14.3151, 14.8816) -> (-13.0753, 14.9331) centre (-13.7222, 15.5587) ccw
  line L12 (-14.3151, 14.8816) -> (-14.5914, 15.1236)
  spline S12 degree 5 poles (-14.5914, 15.1236) (-14.5985, 15.1298) (-14.6129, 15.142) (-14.6348, 15.1598) (-14.665, 15.1823) (-14.7039, 15.209) (-14.7436, 15.2345) (-14.7839, 15.2594) (-14.8246, 15.2839) (-14.8654, 15.3082) (-14.9064, 15.3322) (-14.9477, 15.3558) (-14.9894, 15.379) (-15.0314, 15.4017) (-15.0739, 15.4238) (-15.1168, 15.4454) (-15.1599, 15.4665) (-15.2034, 15.4873) (-15.247, 15.5077) (-15.2909, 15.5279) (-15.335, 15.5477) (-15.3793, 15.5672) (-15.4239, 15.5864) (-15.4687, 15.6052) (-15.5137, 15.6237) (-15.559, 15.6418) (-15.6045, 15.6596) (-15.6502, 15.6771) (-15.696, 15.6943) (-15.7421, 15.7113) (-15.7884, 15.7279) (-15.8348, 15.7442) (-15.8814, 15.7602) (-15.9282, 15.776) (-15.9752, 15.7915) (-16.0224, 15.8066) (-16.0697, 15.8215) (-16.1172, 15.8361) (-16.1649, 15.8505) (-16.2127, 15.8646) (-16.2607, 15.8784) (-16.3088, 15.8919) (-16.3571, 15.9052) (-16.4056, 15.9182) (-16.4541, 15.9309) (-16.5029, 15.9434) (-16.5518, 15.9556) (-16.6008, 15.9676) (-16.65, 15.9793) (-16.6993, 15.9908) (-16.7487, 16.002) (-16.7983, 16.013) (-16.848, 16.0237) (-16.8978, 16.0341) (-16.9478, 16.0444) (-16.9979, 16.0543) (-17.0481, 16.064) (-17.0984, 16.0735) (-17.1489, 16.0828) (-17.1994, 16.0918) (-17.2501, 16.1005) (-17.3009, 16.109) (-17.3519, 16.1173) (-17.4029, 16.1253) (-17.454, 16.1331) (-17.5053, 16.1407) (-17.5567, 16.148) (-17.6081, 16.1551) (-17.6597, 16.162) (-17.7114, 16.1686) (-17.7632, 16.175) (-17.8047, 16.18) (-17.8359, 16.1836) (-17.8567, 16.1859) (-17.8671, 16.1871) knots 0 0 0 0 0 0 0.01428571 0.02857143 0.04285714 0.05714286 0.07142857 0.08571429 0.1 0.11428571 0.12857143 0.14285714 0.15714286 0.17142857 0.18571429 0.2 0.21428571 0.22857143 0.24285714 0.25714286 0.27142857 0.28571429 0.3 0.31428571 0.32857143 0.34285714 0.35714286 0.37142857 0.38571429 0.4 0.41428571 0.42857143 0.44285714 0.45714286 0.47142857 0.48571429 0.5 0.51428571 0.52857143 0.54285714 0.55714286 0.57142857 0.58571429 0.6 0.61428571 0.62857143 0.64285714 0.65714286 0.67142857 0.68571429 0.7 0.71428571 0.72857143 0.74285714 0.75714286 0.77142857 0.78571429 0.8 0.81428571 0.82857143 0.84285714 0.85714286 0.87142857 0.88571429 0.9 0.91428571 0.92857143 0.94285714 0.95714286 0.97142857 0.98571429 1 1 1 1 1 1
  arc A26 (-17.8671, 16.1871) -> (-18.6354, 15.1296) centre (-0.4607, 2.7328) ccw